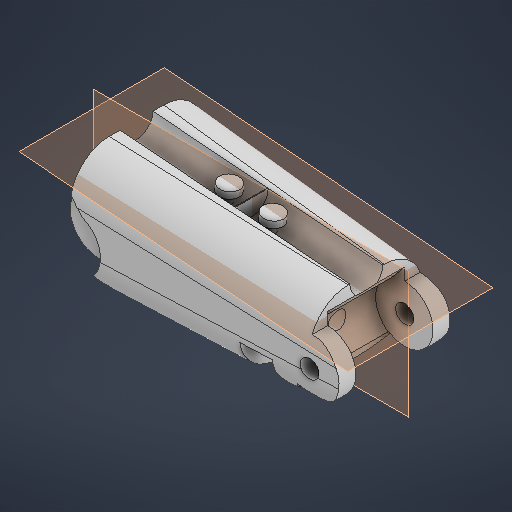
# Autodesk Inventor part: falange1_menique_V12
Saved by Autodesk Inventor 2026.1 (Build 301233020, 233B)
## iProperties
Created: 2026-01-14
Part Number: falange1_menique_V12
Material: Generic
Document SubType Name: Modeling
Designer: user
Density: 1 g/cm^3
Appearance: Default
Author: user
Autodesk Inventor part; units mm, degrees
ref_plane "YZ Plane" through (0, 0, 0) normal (1, 0, 0) x (0, 1, 0)
sketch "Sketch1" plane through (0, 0, 0) normal (0, 0, 1) x (1, 0, 0)
  circle A0 centre (40, 0) radius 1.575
  arc A1 (0, 5) -> (2.8679, -4.0958) centre (0, 0) ccw
  line L0 (0, 5) -> (0, 12.4771)
  arc A2 (37.1751, -4.0343) -> (40, 4.925) centre (40, 0) ccw
  line L1 (40, 4.925) -> (40, 9.275)
  line L2 (2.8679, -4.0958) -> (5.2676, -7.5229)
  line L3 (37.1751, -4.0343) -> (34.7324, -7.5229)
  line L4 (0, 12.4771) -> (40, 9.275)
  line L5 (5.2676, -7.5229) -> (34.7324, -7.5229)
  dimension "d39" = 3.15
  dimension "d46" = 10
  dimension "d57" = 12.4771
  dimension "d131" = 40
  dimension "d132" = 9.85
  dimension "d133" = 4.35
  constraints: 12 end point, 4 point on circle, 3 centre point, 2 coincident, 2 vertical, 1 horizontal
  measures "d39" diameter of A0
  measures "d46" diameter of A1
  measures "d57" distance of L0.end point (0, 0)
  measures "d131" distance of A0.centre point (0, 0)
  measures "d132" diameter of A2
  measures "d133" distance of L1.start L1.end
extrude "Extrusion1" add sketch "Sketch1" along normal mid plane 23
sketch "Sketch3" plane through (0, 0, 11.5) normal (0, 0, 1) x (1, 0, 0)
  circle A0 centre (0, 0) radius 1.575
  circle A1 centre (0, 0) radius 5
  dimension "d49" = 3.15
  dimension "d50" = 10
  constraints: 2 centre point, 2 coincident
  measures "d49" diameter of A0
  measures "d50" diameter of A1
sketch "Sketch4" plane through (0, 0, -11.5) normal (0, 0, -1) x (-1, 0, 0)
  circle A0 centre (0, 0) radius 1.5
  circle A1 centre (0, 0) radius 5
  dimension "d51" = 10
  dimension "d52" = 3
  constraints: 2 centre point, 2 coincident
  measures "d51" diameter of A1
  measures "d52" diameter of A0
extrude "Extrusion3" cut sketch "Sketch3" against normal blind 4.945 contours A0 | A1
extrude "Extrusion4" cut sketch "Sketch4" against normal blind 4.945 contours A0 | A1
sketch "Sketch8" plane through (0, 0, 11.5) normal (0, 0, 1) x (1, 0, 0)
  line L0 (33.6385, -7.5229) -> (28.2676, -7.5229)
  line L1 (28.2676, -7.5229) -> (28.2676, -1.6973)
  line L2 (28.2676, -1.6973) -> (33.6385, -1.6973)
  line L3 (33.6385, -1.6973) -> (33.6385, -7.5229)
  point P0 (0, 0)
  point P1 (36.2741, -7.5229)
  point P2 (5.2676, -7.5229)
  dimension "d67" = 5.8256
  dimension "d90" = 5.3709
  dimension "d186" = 23
  constraints: 8 end point, 2 parallel, 1 horizontal, 1 perpendicular
  measures "d67" distance of L2.end L0.start
  measures "d90" distance of L1.end L2.end
  measures "d186" distance of L0.end point (5.268, -7.523)
extrude "Extrusion5" cut sketch "Sketch8" against normal through all
sketch "Sketch11" plane through (28.2676, -7.5229, 11.5) normal (1, 0, 0) x (0, 0, -1)
  circle A0 centre (11.5, 2.9128) radius 1.5
  point P0 (11.5, 7.5229)
  point P1 (11.5, 0)
  dimension "d75" = 2.9128
  dimension "d76" = 3
  constraints: 1 centre point
  measures "d75" distance of point (11.5, 0) A0.centre
  measures "d76" diameter of A0
extrude "Extrusion8" cut sketch "Sketch11" against normal through all
sketch "Sketch14" plane through (0, 12.4771, -11.5) normal (-1, 0, 0) x (0, 0, 1)
  circle A0 centre (11.5, -12.4771) radius 1.5
  line L0 (0, 0) -> (23, 0) projected
  dimension "d92" = 3
  dimension "d166" = 12.4771
  constraints: 1 centre point, 1 coincident
  measures "d92" diameter of A0
  measures "d166" distance from line of L0 point (11.5, -12.477)
sketch "Sketch15" plane through (0, 0, 0) normal (0, 0, 1) x (1, 0, 0)
  circle A0 centre (0, 0) radius 5
  dimension "d93" = 10
  constraints: 1 centre point, 1 coincident
  measures "d93" diameter of A0
extrude "Extrusion11" cut sketch "Sketch15" along normal mid plane 3.825
extrude "Extrusion12" cut sketch "Sketch3" against normal through all contours A0
sketch "Sketch16" plane through (0, 0, -1.9125) normal (0, 0, 1) x (1, 0, 0)
  point P0 (0, 0)
sketch "Sketch17" plane through (0, 0, 0) normal (0, 0, 1) x (1, 0, 0)
  circle A0 centre (0, 0) radius 1.575 projected
  line L0 (-1.6517, 2.6306) -> (1.4523, 2.7457)
  line L1 (1.4523, 2.7457) -> (3.104, 0.1152)
  line L2 (3.104, 0.1152) -> (1.6517, -2.6306)
  line L3 (1.6517, -2.6306) -> (-1.4523, -2.7457)
  line L4 (-1.4523, -2.7457) -> (-3.104, -0.1152)
  line L5 (-3.104, -0.1152) -> (-1.6517, 2.6306)
  dimension "d102" = 5.38
  constraints: 12 end point, 1 coincident, 13 other
  measures "d102" distance between parallel lines of L3 L0
extrude "Extrusion13" cut sketch "Sketch17" along normal mid plane 8.085 contours A0 | L0 L1 L2 L3 L4 L5
extrude "Extrusion14" cut sketch "Sketch14" against normal through all
sketch "Sketch18" plane through (0, 0, 0) normal (0, 0, 1) x (1, 0, 0)
  circle A0 centre (40, 0) radius 5.075
  circle A1 centre (40, 0) radius 1.575 projected
  point P0 (0, 0)
  dimension "d103" = 10.15
  constraints: 1 centre point
  measures "d103" diameter of A0
extrude "Extrusion15" cut sketch "Sketch18" along normal mid plane 13.41 contours A0 | A1
ref_plane "Work Plane1" through (0, 12.4771, -11.5) normal (0, 1, 0) x (-1, 0, 0)
sketch "Sketch26" plane through (0, 12.4771, -11.5) normal (-1, 0, 0) x (0, 0, 1)
  line L0 (0, 0) -> (23, 0) projected
  circle A0 centre (11.5, 0) radius 2.8604
  point P0 (11.5, -12.4771)
  dimension "d146" = 5.7208
  constraints: 1 centre point, 1 midpoint
  measures "d146" diameter of A0
sketch "Sketch28" plane through (40, 4.925, -11.5) normal (1, 0, 0) x (0, 0, -1)
  line L0 (0, 4.35) -> (-23, 4.35) projected
  circle A0 centre (-11.5, 4.35) radius 2.8604
  point P0 (-11.5, -4.925)
  dimension "d147" = 5.7208
  constraints: 1 centre point, 1 midpoint
  measures "d147" diameter of A0
sketch "Sketch29" plane through (0, 12.4771, 11.5) normal (0.079797, 0.9968111, 0) x (0.9968111, -0.079797, 0)
  line L0 (0, 23) -> (0, 0) projected
  line L1 (0, 11.5) -> (20, 11.5)
  point P0 (0.9956, 11.5)
  dimension "d144" = 20
  constraints: 2 end point, 1 horizontal, 1 midpoint
  measures "d144" distance of L1.start L1.end
sketch "Sketch30" plane through (0, 12.4771, 11.5) normal (0.079797, 0.9968111, 0) x (0.9968111, -0.079797, 0)
  line L0 (40.128, 23) -> (40.128, 0) projected
  line L1 (40.128, 11.5) -> (20.128, 11.5)
  point P0 (0.9956, 11.5)
  dimension "d145" = 20
  constraints: 2 end point, 1 horizontal, 1 midpoint
  measures "d145" distance of L1.start L1.end
sweep "Sweep2" cut profiles "Sketch26" path "Sketch29" path curves L1
sweep "Sweep3" cut profiles "Sketch28" path "Sketch30" path curves L1
ref_plane "Work Plane3" through (-0.2275, 9.6349, 0) normal (0.079797, 0.9968111, 0) x (0.9968111, -0.079797, 0)
sketch "Sketch31" plane through (-0.2275, 9.6349, 0) normal (0.079797, 0.9968111, 0) x (0.9968111, -0.079797, 0)
  line L0 (40.4631, -6.705) -> (40.4631, 6.705) projected
  circle A0 centre (16.24, 0) radius 0.7321
  ellipse E0 centre (0, 0) end of major axis (0, 2.8604) minor radius 0.2283 (0, -2.8604) -> (0, 2.8604) ccw projected
  dimension "d153" = 1.4642
  dimension "d187" = 16.24
  constraints: 1 centre point, 1 other
  measures "d153" diameter of A0
  measures "d187" distance of A0.centre point (0, 0)
extrude "Extrusion23" add sketch "Sketch31" along normal mid plane 3.3575
sketch "Sketch32" plane through (-0.2275, 9.6349, 0) normal (0.079797, 0.9968111, 0) x (0.9968111, -0.079797, 0)
  circle A0 centre (23.888, 0) radius 0.7321
  ellipse E0 centre (40.128, 0) end of major axis (40.128, 2.8604) minor radius 0.2283 (40.128, -2.8604) -> (40.128, 2.8604) ccw projected
  point P0 (-43.9139, -2.8604)
  point P1 (-43.9139, 2.8604)
  dimension "d157" = 1.4642
  dimension "d188" = 16.24
  constraints: 1 centre point, 1 other
  measures "d157" diameter of A0
  measures "d188" distance of point (40.128, 0) A0.centre
extrude "Extrusion24" add sketch "Sketch32" along normal mid plane 3.3575
sketch "Sketch33" plane through (23.7182, 9.4021, 0) normal (0.079797, 0.9968111, 0) x (0.9968111, -0.079797, 0)
  circle A0 centre (0, 0) radius 0.7321 projected
  circle A1 centre (0, 0) radius 1.774
  point P0 (-22.8923, 0)
  point P1 (-0.6816, 0.2673)
  point P2 (0.6816, 0.2673)
  dimension "d160" = 3.548
  constraints: 1 centre point, 1 coincident
  measures "d160" diameter of A1
extrude "Extrusion25" add sketch "Sketch33" along normal up to surface (1.1725 mm away) contours A0 | A1
sketch "Sketch34" plane through (16.0946, 10.0124, 0) normal (0.079797, 0.9968111, 0) x (0.9968111, -0.079797, 0)
  circle A0 centre (0, 0) radius 0.7321 projected
  circle A1 centre (0, 0) radius 1.774
  point P0 (-15.2444, 0)
  dimension "d163" = 3.548
  constraints: 1 centre point, 1 coincident
  measures "d163" diameter of A1
extrude "Extrusion26" add sketch "Sketch34" along normal up to surface (1.1725 mm away) contours A0 | A1
chamfer "Chamfer1" distance 2 angle 45 1 edges at (40, 5.075, 0)
chamfer "Chamfer2" distance 2 angle 45 2 edges at (0, 5, -9.0275) (0, 5, 9.0275)
sketch "Sketch35" plane through (33.6385, -7.5229, 11.5) normal (-1, 0, 0) x (0, 0, 1)
  line L0 (0, 5.8256) -> (-23, 5.8256) projected
  line L1 (0, 5.8256) -> (0, 0) projected
  line L2 (-23, 5.8256) -> (0, 5.8256)
  circle A0 centre (-11.5, 1.997) radius 1
  point P0 (-11.5, 7.5229)
  dimension "d173" = 2
  constraints: 2 end point, 1 centre point, 1 perpendicular
  measures "d173" diameter of A0
sketch "Sketch38" plane through (5.2676, -7.5229, -11.5) normal (0, -1, 0) x (1, 0, 0)
  line L0 (-5.2676, 23) -> (-5.2676, 18.055) projected
  line L1 (-5.2676, 23) -> (43.4544, 21)
  line L2 (43.4544, 21) -> (43.4544, 11.5)
  line L3 (39.6574, 18.205) -> (39.6574, 23) projected
  line L4 (-40.661, 11.5) -> (57.4736, 11.5) projected
  line L5 (-3.6158, 13.4125) -> (-3.6158, 15.5425) projected
  line L6 (-5.2676, 0) -> (43.4544, 2)
  line L7 (43.4544, 2) -> (43.4544, 11.5)
  line L8 (-5.2676, 23) -> (-26.6418, 23)
  line L9 (-26.6418, 23) -> (-26.6418, 11.5)
  line L10 (-5.2676, 0) -> (-26.6418, 0)
  line L11 (-26.6418, 0) -> (-26.6418, 11.5)
  point P0 (-5.2676, 11.5)
  dimension "d179" = 9.5
  constraints: 16 end point, 3 symmetric about line, 2 perpendicular, 2 point on line, 1 horizontal, 1 parallel
  measures "d179" distance of L1.end L2.end
extrude "Extrusion27" cut sketch "Sketch38" against normal through all keep common part
fillet "Fillet1" radius 6.7625 2 edges at (20, 10.876, 10.679) (20, 10.876, -10.679)
fillet "Fillet2" radius 6.7625 2 edges at (16.7676, -7.5229, 10.8117) (16.7676, -7.5229, -10.8117)
extrude "Extrusion28" cut sketch "Sketch35" against normal blind 10
equation "\"d39\" = diametroDentroUnion + tolerancia"
equation "\"d46\" = diametroFueraUnion"
equation "\"d132\" = diametroFueraUnion - tolerancia"
equation "\"d49\" = diametroDentroUnion + tolerancia"
equation "\"d50\" = diametroFueraUnion"
equation "\"d51\" = diametroFueraUnion"
equation "\"d52\" = diametroDentroUnion"
equation "\"d93\" = diametroFueraUnion"
equation "\"d103\" = diametroFueraUnion + tolerancia"
equation "\"diametroDentroUnion\" = 3"
equation "\"diametroFueraUnion\" = 10"
equation "\"tolerancia\" = 0.15"
body "Solid1"
